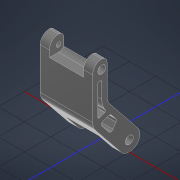
# Autodesk Inventor part: Swing-Arm B
Saved by Autodesk Inventor 2022.2 (Build 262287010, 287A)
## iProperties
Created: 2022-03-22
Part Number: Swing-Arm B
Material: ABS-Kunststoff
Document SubType Name: Modeling
Designer: sleib
Density: 1.06 g/cm^3
Appearance: Glatt - Schwarz
Author: sleib
Autodesk Inventor part; units mm, degrees
ref_plane "YZ Plane" through (0, 0, 0) normal (1, 0, 0) x (0, 1, 0)
ref_plane "XZ Plane" through (0, 0, 0) normal (0, 1, 0) x (-1, 0, 0)
ref_plane "XY Plane" through (0, 0, 0) normal (0, 0, 1) x (1, 0, 0)
sketch "SwingArm B" plane through (0, 0, 0) normal (0, 0, 1) x (1, 0, 0)
  arc A0 (25.4839, 28) -> (19.2029, 25.7813) centre (25.4839, 18) ccw
  arc A1 (37.33, 17) -> (31.049, 14.7813) centre (37.33, 7) ccw
  circle A2 centre (0, 0) radius 8 construction
  arc A3 (-5.0248, 6.2251) -> (5.0248, -6.2251) centre (0, 0) ccw
  line L0 (31.049, 14.7813) -> (5.0248, -6.2251)
  line L1 (19.2029, 25.7813) -> (-5.0248, 6.2251)
  line L2 (57, 28) -> (25.4839, 28)
  line L3 (60, 17) -> (37.33, 17)
  circle A4 centre (57, 21) radius 7 construction
  arc A5 (64, 21) -> (57, 28) centre (57, 21) ccw
  arc A6 (60, 17) -> (64, 21) centre (60, 21) ccw
  circle A7 centre (0, 0) radius 1.7
  circle A8 centre (57, 21) radius 1.7
  line L4 (57, 21) -> (26.0163, 21) construction
  line L5 (26.0163, 21) -> (0, 0) construction
  line L6 (22.6557, 20.0016) -> (24.0687, 16.0016)
  line L7 (23.4391, 13.7792) -> (19.1745, 10.3369)
  line L8 (16.8693, 10.1904) -> (13.2575, 12.4154)
  line L9 (13.0503, 15.6745) -> (19.5137, 20.8917)
  arc A9 (22.6557, 20.0016) -> (19.5137, 20.8917) centre (20.7699, 19.3355) ccw
  arc A10 (23.4391, 13.7792) -> (24.0687, 16.0016) centre (22.1829, 15.3355) ccw
  arc A11 (16.8693, 10.1904) -> (19.1745, 10.3369) centre (17.9183, 11.8932) ccw
  arc A12 (13.0503, 15.6745) -> (13.2575, 12.4154) centre (14.3065, 14.1182) ccw
  line L10 (22.1532, 27.429) -> (27.6033, 12) construction
  line L11 (37.33, 21) -> (60, 21) construction
  arc A13 (60, 21) -> (57, 24) centre (57, 21) ccw construction
  line L12 (57, 24) -> (25.4839, 24) construction
  arc A14 (25.4839, 24) -> (21.7153, 22.6688) centre (25.4839, 18) ccw construction
  line L13 (21.7153, 22.6688) -> (-2.5124, 3.1125) construction
  arc A15 (-2.5124, 3.1125) -> (2.5124, -3.1125) centre (0, 0) ccw construction
  line L14 (2.5124, -3.1125) -> (28.5366, 17.8939) construction
  arc A16 (37.33, 21) -> (28.5366, 17.8939) centre (37.33, 7) ccw construction
  line L15 (49.9641, 21.75) -> (50.2223, 22.75)
  line L16 (27.3731, 18.6564) -> (25.9565, 22.6669)
  line L17 (48.9958, 21) -> (37.33, 21)
  line L18 (49.254, 24) -> (26.8994, 24)
  arc A17 (37.33, 21) -> (28.917, 18.1902) centre (37.33, 7) ccw
  arc A18 (27.3731, 18.6564) -> (28.917, 18.1902) centre (28.316, 18.9895) ccw
  arc A19 (26.8994, 24) -> (25.9565, 22.6669) centre (26.8994, 23) ccw
  arc A20 (50.2223, 22.75) -> (49.254, 24) centre (49.254, 23) ccw
  arc A21 (48.9958, 21) -> (49.9641, 21.75) centre (48.9958, 22) ccw
  line L19 (16.282, 18.2831) -> (21.3068, 12.0581) construction
  line L20 (11.494, 14.4183) -> (16.5188, 8.1932) construction
  dimension "d0" = 3.4
  dimension "d1" = 3.4
  dimension "d2" = 57
  dimension "d3" = 21
  dimension "d4" = 141.09
  dimension "d5" = 4
  dimension "d6" = 7
  dimension "d7" = 4
  dimension "d10" = 10
  dimension "d11" = 10
  dimension "d13" = 2
  dimension "d14" = 2
  dimension "d42" = 16
  dimension "d43" = 4
  dimension "d45" = 1
  dimension "d46" = 4
  dimension "d49" = 18
  measures "d0" diameter of A7
  measures "d1" diameter of A8
  measures "d2" horizontal distance of L5.end L4.start
  measures "d3" vertical distance of L5.end L4.start
  measures "d4" angle of L5 L4
  measures "d5" distance from line of L3 L4.start
  measures "d6" distance from line of L4.start L2
  measures "d7" radius of A6
  measures "d10" radius of A1
  measures "d11" radius of A0
  measures "d13" radius of A9
  measures "d14" radius of A10
  measures "d42" diameter of A2
  measures "d43" distance between parallel lines of L3 L11
  measures "d45" radius of A20
  measures "d46" distance between parallel lines of L6 L16
  measures "d49" distance from line of point (0, 0) L20
sketch "Skizze1" plane through (0, 0, 0) normal (1, 0, 0) x (0, 1, 0)
  circle A0 centre (0, 0) radius 18
  arc A1 (52, 21) -> (54, 17) centre (57, 21) ccw
  line L0 (52, 21) -> (52, 28)
  arc A2 (25.4839, 28) -> (19.2029, 25.7813) centre (25.4839, 18) ccw
  arc A3 (37.33, 17) -> (31.049, 14.7813) centre (37.33, 7) ccw
  circle A4 centre (0, 0) radius 8 construction
  arc A5 (-5.0248, 6.2251) -> (5.0248, -6.2251) centre (0, 0) ccw
  line L1 (31.049, 14.7813) -> (5.0248, -6.2251)
  line L2 (19.2029, 25.7813) -> (-5.0248, 6.2251)
  line L3 (57, 28) -> (25.4839, 28)
  line L4 (60, 17) -> (37.33, 17)
  circle A6 centre (57, 21) radius 7 construction
  arc A7 (64, 21) -> (57, 28) centre (57, 21) ccw
  arc A8 (60, 17) -> (64, 21) centre (60, 21) ccw
  circle A9 centre (0, 0) radius 1.7
  circle A10 centre (57, 21) radius 1.7
  line L5 (57, 21) -> (26.0163, 21) construction
  line L6 (26.0163, 21) -> (0, 0) construction
  line L7 (22.6557, 20.0016) -> (24.0687, 16.0016)
  line L8 (23.4391, 13.7792) -> (19.1745, 10.3369)
  line L9 (16.8693, 10.1904) -> (13.2575, 12.4154)
  line L10 (13.0503, 15.6745) -> (19.5137, 20.8917)
  arc A11 (22.6557, 20.0016) -> (19.5137, 20.8917) centre (20.7699, 19.3355) ccw
  arc A12 (23.4391, 13.7792) -> (24.0687, 16.0016) centre (22.1829, 15.3355) ccw
  arc A13 (16.8693, 10.1904) -> (19.1745, 10.3369) centre (17.9183, 11.8932) ccw
  arc A14 (13.0503, 15.6745) -> (13.2575, 12.4154) centre (14.3065, 14.1182) ccw
  line L11 (22.1532, 27.429) -> (27.6033, 12) construction
  line L12 (37.33, 21) -> (60, 21) construction
  arc A15 (60, 21) -> (57, 24) centre (57, 21) ccw construction
  line L13 (57, 24) -> (25.4839, 24) construction
  arc A16 (25.4839, 24) -> (21.7153, 22.6688) centre (25.4839, 18) ccw construction
  line L14 (21.7153, 22.6688) -> (-2.5124, 3.1125) construction
  arc A17 (-2.5124, 3.1125) -> (2.5124, -3.1125) centre (0, 0) ccw construction
  line L15 (2.5124, -3.1125) -> (28.5366, 17.8939) construction
  arc A18 (37.33, 21) -> (28.5366, 17.8939) centre (37.33, 7) ccw construction
  line L16 (49.9641, 21.75) -> (50.2223, 22.75)
  line L17 (27.3731, 18.6564) -> (25.9565, 22.6669)
  line L18 (48.9958, 21) -> (37.33, 21)
  line L19 (49.254, 24) -> (26.8994, 24)
  arc A19 (37.33, 21) -> (28.917, 18.1902) centre (37.33, 7) ccw
  arc A20 (27.3731, 18.6564) -> (28.917, 18.1902) centre (28.316, 18.9895) ccw
  arc A21 (26.8994, 24) -> (25.9565, 22.6669) centre (26.8994, 23) ccw
  arc A22 (50.2223, 22.75) -> (49.254, 24) centre (49.254, 23) ccw
  arc A23 (48.9958, 21) -> (49.9641, 21.75) centre (48.9958, 22) ccw
  line L20 (16.282, 18.2831) -> (21.3068, 12.0581) construction
  line L21 (11.494, 14.4183) -> (16.5188, 8.1932) construction
  point P0 (17.5718, 3.9027)
  point P1 (7.5222, 16.3529)
  point P2 (-5.0248, 6.2251)
  point P3 (5.0248, -6.2251)
  point P4 (54, 17)
  dimension "d40" = 36
  dimension "d51" = 10
  constraints: 2 centre point, 2 end point, 2 point on circle, 1 tangent, 1 vertical, 6 other
  measures "d40" diameter of A0
  measures "d51" diameter of A1
extrude "Extrusion1" add sketch "Skizze1" along normal mid plane 40 contours L1 A5 L2 A0 | A0 L2 A2 L3 L0 A1 L4 A3 L1 | A1 L0 L3 A7 A8 L4 picked at (1.0334, 8.0558)
extrude "Extrusion6" cut sketch "Skizze1" along normal mid plane 26 contours L1 A5 L2 A0 | A1 L0 L3 A7 A8 L4 picked at (1.0334, 8.0558)
sketch "Skizze4" plane through (20, 0, 0) normal (1, 0, 0) x (0, 0, -1)
  circle A0 centre (0, 0) radius 3
  circle A1 centre (-21, 57) radius 1.7 projected
  circle A2 centre (-21, 57) radius 3
  dimension "d27" = 6
  dimension "d33" = 6
  constraints: 2 centre point, 2 coincident
  measures "d27" diameter of A0
  measures "d33" diameter of A2
extrude "Extrusion4" cut sketch "Skizze4" against normal blind 4
sketch "Skizze5" plane through (-20, 0, 0) normal (-1, 0, 0) x (0, 0, 1)
  line L0 (2.75, 1.5877) -> (2.75, -1.5877)
  line L1 (2.75, -1.5877) -> (0, -3.1754)
  line L2 (0, -3.1754) -> (-2.75, -1.5877)
  line L3 (-2.75, -1.5877) -> (-2.75, 1.5877)
  line L4 (-2.75, 1.5877) -> (0, 3.1754)
  line L5 (0, 3.1754) -> (2.75, 1.5877)
  circle A0 centre (21, 57) radius 1.7 projected
  line L6 (23.75, 58.5877) -> (23.75, 55.4123)
  line L7 (23.75, 55.4123) -> (21, 53.8246)
  line L8 (21, 53.8246) -> (18.25, 55.4123)
  line L9 (18.25, 55.4123) -> (18.25, 58.5877)
  line L10 (18.25, 58.5877) -> (21, 60.1754)
  line L11 (21, 60.1754) -> (23.75, 58.5877)
  line L12 (17, 60) -> (17, 37.33) projected
  point P0 (0, 0)
  point P1 (0, 0)
  dimension "d30" = 5.5
  dimension "d34" = 5.5
  constraints: 24 end point, 2 coincident, 2 parallel, 26 other
  measures "d30" distance between parallel lines of L2 L5
  measures "d34" distance between parallel lines of L6 L9
extrude "Extrusion5" cut sketch "Skizze5" against normal blind 4
